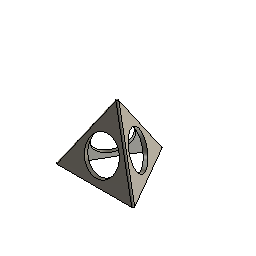
Day15tetrahedron (Autodesk Fusion 360 design; units mm, degrees)
part number: 2025-12-01-17-36-41-826
Autodesk Fusion 360 part; units mm, degrees
sketch "Sketch1" plane through (0, 0, 0) normal (0, 0, 1) x (1, 0, 0)
  line L0 (0, 0) -> (30, 51.9615)
  line L1 (30, 51.9615) -> (60, 0)
  line L2 (60, 0) -> (0, 0)
  dimension "d3" = 60
  constraint coincident L0.start L2.end
  constraint horizontal L2
  constraint equal L0 L1
  constraint equal L0 L2
  measures "d3" distance of L0.start L0.end
ref_plane "WorkPlane1" through (30, 25.9808, 50) normal (0, 0, 1) x (1, 0, 0)
sketch "Sketch2" plane through (0, 0, 50) normal (0, 0, 1) x (1, 0, 0)
  line L0 (0, 0) -> (30, 51.9615)
  line L1 (30, 51.9615) -> (60, 0)
  line L2 (60, 0) -> (0, 0)
  line L3 (0, 0) -> (45, 25.9808)
  line L4 (30, 51.9615) -> (30, 0)
  point P0 (30, 17.3205)
  constraint coincident L0.start L2.end
  constraint midpoint L1 L3.end
  constraint coincident L0.end L1.start
  constraint midpoint L2 L4.end
  constraint coincident L3 P0
  constraint coincident L4 P0
loft "Loft1" add profiles "Sketch1" section 1 section 2 point at (30, 17.3205, 50)
shell "Shell1" thickness 2.5 removed faces 1 at (30, 17.3205, 0)
sketch "Sketch3" plane through (0, 0, 0) normal (0, 1, 0) x (1, 0, 0)
  line L0 (0, 0) -> (60, 0)
  line L1 (60, 0) -> (30, -50)
  line L2 (30, -50) -> (0, 0)
  line L3 (0, 0) -> (45, -25)
  line L4 (30, -50) -> (30, 0)
  circle A0 centre (30, -16.6667) radius 12.5
  dimension "d6" = 25
  constraint coincident L0.start L2.end
  constraint midpoint L1 L3.end
  constraint coincident L1.end L2.start
  constraint midpoint L0 L4.end
  constraint coincident L4 A0.centre
  constraint coincident L3 A0.centre
  measures "d6" diameter of A0
extrude "Extrude1" cut sketch "Sketch3" along normal up to surface contours L3 L4 A0 | L3 L4 A0 | L3 L4 A0 | L3 L4 A0 end surface through (60, 2.3623, -0.8183) normal (0, 0.944911, -0.327327) offset 0
pattern_circular "C-Pattern1" count 3 over 360 about axis through (30, 17.3205, 75) along (0, 0, -1) of 1 faces at (41.2562, 9.4162, 22.1025)
fillet "Fillet1" radius 1 3 edges at (45, 8.6603, 25) (15, 8.6603, 25) (30, 34.641, 25)
